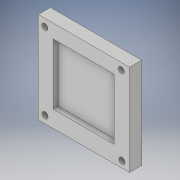
# Autodesk Inventor part: carromboard15cm
Saved by Autodesk Inventor 2019 (Build 230136000, 136)
## iProperties
Created: 2020-03-04
Part Number: carromboard15cm
Material: Generic
Document SubType Name: Modeling
Designer: Hp
Density: 1 g/cm^3
Appearance: Default
Author: Hp
Autodesk Inventor part; units mm, degrees
ref_plane "YZ Plane" through (0, 0, 0) normal (1, 0, 0) x (0, 1, 0)
ref_plane "XZ Plane" through (0, 0, 0) normal (0, 1, 0) x (-1, 0, 0)
ref_plane "XY Plane" through (0, 0, 0) normal (0, 0, 1) x (1, 0, 0)
sketch "Sketch1" plane through (0, 0, 0) normal (0, 0, 1) x (1, 0, 0)
  line L0 (0, 0) -> (150, 0)
  line L1 (150, 0) -> (150, -150)
  line L2 (150, -150) -> (0, -150)
  line L3 (0, -150) -> (0, 0)
  dimension "d0" = 150
  dimension "d1" = 150
  constraints: 8 end point, 2 parallel, 1 horizontal, 1 perpendicular
  measures "d0" distance of L1.end L2.end
  measures "d1" distance of L0.end L1.end
extrude "Extrusion1" add sketch "Sketch1" along normal blind 20
sketch "Sketch2" plane through (0, 0, 20) normal (0, 0, 1) x (1, 0, 0)
  line L0 (24.5154, -22.5096) -> (124.5154, -22.5096)
  line L1 (124.5154, -22.5096) -> (124.5154, -122.5096)
  line L2 (124.5154, -122.5096) -> (24.5154, -122.5096)
  line L3 (24.5154, -122.5096) -> (24.5154, -22.5096)
  point P0 (0, 0)
  dimension "d4" = 100
  dimension "d5" = 100
  constraints: 8 end point, 2 parallel, 1 horizontal, 1 perpendicular
  measures "d4" distance of L1.end L2.end
  measures "d5" distance of L0.end L1.end
extrude "Extrusion2" cut sketch "Sketch2" against normal blind 8
sketch "Sketch3" plane through (0, 0, 20) normal (0, 0, 1) x (1, 0, 0)
  point P0 (0, 0)
  point P1 (10.7394, -12.154)
  point P2 (136.4315, -10.9415)
  point P3 (137.6439, -139.4626)
  point P4 (11.1436, -137.846)
hole "Hole1" at (10.7394, -12.154, 20) at (136.4315, -10.9415, 20) at (137.6439, -139.4626, 20) at (11.1436, -137.846, 20) direction (0, 0, -1) diameter 10 depth 30 tip angle 118
body "Solid1"
